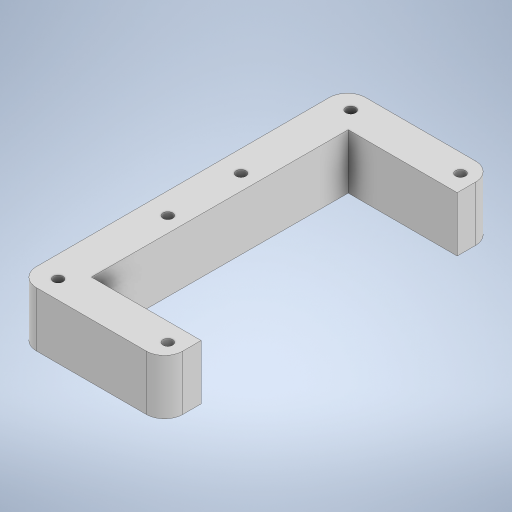
# Autodesk Inventor part: Swerve_BH
Saved by Autodesk Inventor 2024 (Build 280153000, 153)
## iProperties
Created: 2023-08-14
Part Number: Swerve_BH
Material: Generic
Document SubType Name: Modeling
Designer: s137416
Density: 1 g/cm^3
Appearance: Default
Author: s137416
Autodesk Inventor part; units mm, degrees
ref_plane "YZ Plane" through (0, 0, 0) normal (1, 0, 0) x (0, 1, 0)
ref_plane "XZ Plane" through (0, 0, 0) normal (0, 1, 0) x (-1, 0, 0)
ref_plane "XY Plane" through (0, 0, 0) normal (0, 0, 1) x (1, 0, 0)
sketch "Sketch1" plane through (0, 0, 0) normal (0, 1, 0) x (-1, 0, 0)
  line L0 (-50.8, 114.3) -> (50.8, 114.3)
  line L1 (50.8, 114.3) -> (50.8, -114.3)
  line L2 (50.8, -114.3) -> (-50.8, -114.3)
  line L3 (-50.8, -114.3) -> (-50.8, 114.3)
  line L4 (-50.8, 114.3) -> (50.8, -114.3) construction
  line L5 (50.8, 114.3) -> (-50.8, -114.3) construction
  line L6 (-50.8, 88.9) -> (25.4, 88.9)
  line L7 (25.4, 88.9) -> (24.8543, -88.9)
  line L8 (24.8543, -88.9) -> (-50.8, -88.9)
  point P0 (0, 0)
  dimension "d0" = 101.6
  dimension "d1" = 228.6
  dimension "d2" = 76.2
  dimension "d3" = 25.4
  dimension "d4" = 25.4
  constraints: 18 end point, 3 perpendicular, 2 midpoint, 2 parallel, 2 point on line, 1 horizontal
  measures "d0" distance of L1.end L2.end
  measures "d1" distance of L0.end L1.end
  measures "d2" distance of L6.start L6.end
  measures "d3" distance between parallel lines of L0 L6
  measures "d4" distance from line of L2 L7.end
extrude "Extrusion1" add sketch "Sketch1" along normal blind 38.1 contours L0 L1 L2 L3 L8 L7 L6
fillet "Fillet1" radius 12.7 4 edges at (50.8, 19.05, 114.3) (-50.8, 19.05, 114.3) (-50.8, 19.05, -114.3) (50.8, 19.05, -114.3)
sketch "Sketch2" plane through (0, 38.1, 0) normal (0, 1, 0) x (1, 0, 0)
  line L0 (-38.1, -114.3) -> (38.1, -114.3) projected
  circle A0 centre (-35.8052, -101.6) radius 3.3782
  circle A1 centre (40.3948, -101.6) radius 3.3782
  circle A2 centre (-35.8052, -25.4) radius 3.3782
  circle A3 centre (-35.8052, 25.4) radius 3.3782
  circle A4 centre (-35.8052, 101.6) radius 3.3782
  circle A5 centre (40.3948, 101.6) radius 3.3782
  point P0 (0, 0)
  dimension "d8" = 12.7
  dimension "d9" = 76.2
  dimension "d10" = 127
  dimension "d11" = 203.2
  dimension "d12" = 76.2
  dimension "d13" = 6.7564
  dimension "d14" = 6.7564
  dimension "d15" = 6.7564
  dimension "d16" = 6.7564
  dimension "d17" = 6.7564
  dimension "d18" = 6.7564
  constraints: 6 centre point, 6 coincident
  measures "d8" distance from line of L0 point (-35.805, -101.6)
  measures "d9" distance of point (-35.805, -25.4) point (-35.805, -101.6)
  measures "d10" distance of point (-35.805, 25.4) point (-35.805, -101.6)
  measures "d11" distance of point (-35.805, 101.6) point (-35.805, -101.6)
  measures "d12" distance of point (40.395, -101.6) point (-35.805, -101.6)
  measures "d13" diameter of A0
  measures "d14" diameter of A1
  measures "d15" diameter of A2
  measures "d16" diameter of A3
  measures "d17" diameter of A4
  measures "d18" diameter of A5
extrude "Extrusion2" cut sketch "Sketch2" against normal through all
body "Solid1"
